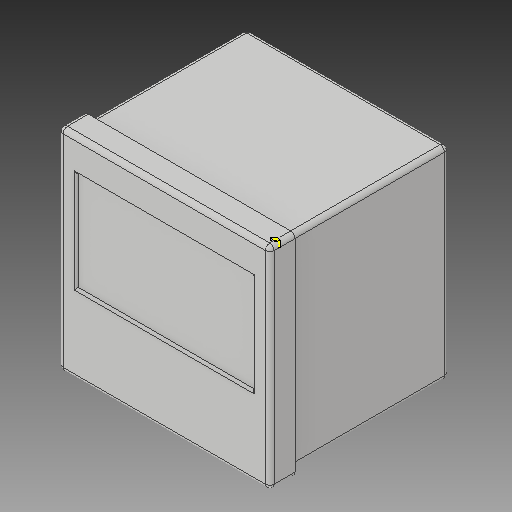
# Autodesk Inventor part: EM20
Saved by Autodesk Inventor 2019.3 (Build 233278000, 278)
## iProperties
Created: 2018-12-14
Part Number: EM20
Material: Типовые
Document SubType Name: Modeling
Designer: A.Vlaschuk
Density: 1 g/cm^3
Appearance: По умолчанию
Author: A.Vlaschuk
Autodesk Inventor part; units mm, degrees
ref_plane "YZ Plane" through (0, 0, 0) normal (1, 0, 0) x (0, 1, 0)
ref_plane "XZ Plane" through (0, 0, 0) normal (0, 1, 0) x (-1, 0, 0)
ref_plane "XY Plane" through (0, 0, 0) normal (0, 0, 1) x (1, 0, 0)
sketch "Эскиз1" plane through (0, 0, 0) normal (0, 0, 1) x (1, 0, 0)
  line L0 (0, 0) -> (-96, 0)
  line L1 (-96, 0) -> (-96, -96)
  line L2 (-96, -96) -> (0, -96)
  line L3 (0, -96) -> (0, 0)
  dimension "d0" = 96
  dimension "d1" = 96
  constraints: 8 end point, 2 parallel, 1 horizontal, 1 perpendicular
  measures "d0" distance of L2.end L1.end
  measures "d1" distance of L1.end L0.end
extrude "Выдавливание1" add sketch "Эскиз1" along normal blind 11.5
fillet "Сопряжение1" radius 2 8 edges at (-48, 0, 11.5) (-96, -48, 11.5) (-96, 0, 5.75) (-96, -96, 5.75) (-48, -96, 11.5) (0, -48, 11.5) (0, -96, 5.75) (0, 0, 5.75)
sketch "Эскиз2" plane through (0, 0, 0) normal (0, 0, -1) x (-1, 0, 0)
  line L0 (2, -2) -> (94, -2)
  line L1 (94, -2) -> (94, -94)
  line L2 (94, -94) -> (2, -94)
  line L3 (2, -94) -> (2, -2)
  line L4 (18.852, -2) -> (35.4089, -2)
  line L5 (0, -94) -> (0, -2) projected
  line L6 (2, 0) -> (94, 0) projected
  point P0 (0, 0)
  dimension "d5" = 92
  dimension "d6" = 92
  dimension "d7" = 2
  dimension "d8" = 2
  constraints: 10 end point, 2 horizontal, 2 parallel, 1 perpendicular, 1 point on line
  measures "d5" distance of L1.end L2.end
  measures "d6" distance of L0.end L1.end
  measures "d7" distance between parallel lines of L5 L3
  measures "d8" distance between parallel lines of L6 L0
extrude "Выдавливание2" add sketch "Эскиз2" along normal blind 72
fillet "Сопряжение2" radius 2 8 edges at (-2, -2, -36) (-48, -2, -72) (-2, -48, -72) (-2, -94, -36) (-48, -94, -72) (-94, -94, -36) (-94, -48, -72) (-94, -2, -36)
sketch "Эскиз4" plane through (0, 0, 11.5) normal (0, 0, 1) x (1, 0, 0)
  line L0 (-88, -15) -> (-8, -15)
  line L1 (-8, -15) -> (-8, -60)
  line L2 (-8, -60) -> (-88, -60)
  line L3 (-88, -60) -> (-88, -15)
  line L4 (0, -94) -> (0, -2) projected
  line L5 (-2, 0) -> (-94, 0) projected
  point P0 (0, 0)
  dimension "d15" = 45
  dimension "d16" = 80
  dimension "d17" = 8
  dimension "d21" = 15
  constraints: 8 end point, 2 parallel, 1 horizontal, 1 perpendicular
  measures "d15" distance of L0.end L1.end
  measures "d16" distance of L0.start L0.end
  measures "d17" distance between parallel lines of L4 L1
  measures "d21" distance between parallel lines of L5 L0
extrude "Выдавливание4" cut sketch "Эскиз4" against normal blind 1
fillet "Сопряжение3" radius 1 4 edges at (-8, -37.5, 11.5) (-48, -60, 11.5) (-48, -15, 11.5) (-88, -37.5, 11.5)
